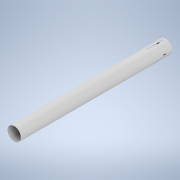
# Autodesk Inventor part: Body Tube
Saved by Autodesk Inventor 2022 (Build 260153000, 153)
## iProperties
Created: 2021-10-30
Part Number: Body Tube
Material: Generic
Document SubType Name: Modeling
Designer: Ryan
Density: 1 g/cm^3
Appearance: Default
Author: Ryan
Autodesk Inventor part; units mm, degrees
ref_plane "YZ Plane" through (0, 0, 0) normal (1, 0, 0) x (0, 1, 0)
ref_plane "XZ Plane" through (0, 0, 0) normal (0, 1, 0) x (-1, 0, 0)
ref_plane "XY Plane" through (0, 0, 0) normal (0, 0, 1) x (1, 0, 0)
sketch "Sketch1" plane through (0, 0, 0) normal (1, 0, 0) x (0, 1, 0)
  line L0 (0, 0) -> (-38.1, 0)
  line L1 (-38.1, 0) -> (-38.1, 864)
  line L2 (-38.1, 864) -> (0, 864)
  line L3 (0, 864) -> (0, 0)
  dimension "d0" = 38.1
  dimension "d1" = 864
  constraints: 8 end point, 2 parallel, 1 horizontal, 1 perpendicular
  measures "d0" distance of L1.end L2.end
  measures "d1" distance of L0.end L1.end
revolve "Revolution1" add sketch "Sketch1" angle 360 about axis through (0, 0, 864) along (0, 0, -1)
sketch "Sketch2" plane through (0, 0, 864) normal (0, 0, 1) x (1, 0, 0)
  circle A0 centre (0, 0) radius 36.83
  circle A1 centre (0, 0) radius 38.1 projected
  dimension "d3" = 1.27
  constraints: 1 centre point, 1 coincident
  measures "d3" radial gap between concentric circles of A1 A0
extrude "Extrusion1" cut sketch "Sketch2" against normal through all contours A0
sketch "Sketch3" plane through (0, 0, 0) normal (1, 0, 0) x (0, 1, 0)
  line L0 (0, 0) -> (0, 12.7)
  line L1 (0, 12.7) -> (3.175, 12.7)
  line L2 (3.175, 12.7) -> (3.175, 107.95)
  line L3 (3.175, 107.95) -> (0, 107.95)
  line L4 (0, 12.7) -> (-3.175, 12.7)
  line L5 (-3.175, 12.7) -> (-3.175, 107.95)
  line L6 (-3.175, 107.95) -> (0, 107.95)
  dimension "d6" = 12.7
  dimension "d10" = 3.175
  dimension "d11" = 95.25
  dimension "d12" = 3.175
  constraints: 14 end point, 2 horizontal, 2 parallel, 2 perpendicular, 1 vertical
  measures "d6" distance of L0.start L0.end
  measures "d10" distance of L3.end L2.end
  measures "d11" distance of L1.end L2.end
  measures "d12" distance of L5.end L6.end
extrude "Extrusion2" cut sketch "Sketch3" along normal through all both and the other way through all
sketch "Sketch4" plane through (0, 0, 0) normal (0, 1, 0) x (-1, 0, 0)
  line L0 (0, 0) -> (0, 12.7)
  line L1 (0, 12.7) -> (3.175, 12.7)
  line L2 (3.175, 12.7) -> (3.175, 107.95)
  line L3 (3.175, 107.95) -> (0, 107.95)
  line L4 (0, 12.7) -> (-3.175, 12.7)
  line L5 (-3.175, 12.7) -> (-3.175, 107.95)
  line L6 (-3.175, 107.95) -> (0, 107.95)
  dimension "d15" = 12.7
  dimension "d16" = 3.175
  dimension "d17" = 95.25
  dimension "d18" = 3.175
  dimension "d19" = 95.25
  constraints: 14 end point, 2 horizontal, 2 parallel, 2 perpendicular, 1 vertical
  measures "d15" distance of L0.start L0.end
  measures "d16" distance of L3.end L2.end
  measures "d17" distance of L1.end L2.end
  measures "d18" distance of L5.end L6.end
  measures "d19" distance of L4.end L5.end
extrude "Extrusion3" cut sketch "Sketch4" along normal through all both and the other way through all
body "Solid1"
